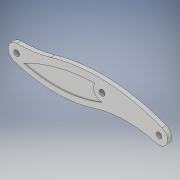
# Autodesk Inventor part: legB_mini
Saved by Autodesk Inventor 2017 (Build 210142000, 142)
## iProperties
Created: 2016-08-26
Part Number: legB_mini
Material: Generic
Document SubType Name: Modeling
Designer: Nic
Density: 1 g/cm^3
Appearance: Default
Author: Nic
Autodesk Inventor part; units mm, degrees
ref_plane "YZ Plane" through (0, 0, 0) normal (1, 0, 0) x (0, 1, 0)
ref_plane "XZ Plane" through (0, 0, 0) normal (0, 1, 0) x (-1, 0, 0)
sketch "Sketch1" plane through (0, 0, 0) normal (0, 0, 1) x (1, 0, 0)
  circle A0 centre (0, 0) radius 1
  circle A1 centre (50, 0) radius 1
  circle A2 centre (30, 3) radius 1
  circle A3 centre (0, 0) radius 3 construction
  circle A4 centre (50, 0) radius 3 construction
  circle A5 centre (30, 3) radius 3 construction
  arc A6 (0, 3) -> (-0.9702, -2.8388) centre (0, 0) ccw
  arc A7 (-0.9702, -2.8388) -> (27.1592, -3.1605) centre (13.5833, 39.7428) ccw
  arc A8 (51.1182, 2.7838) -> (11.9578, 4.708) centre (28.755, -52.8928) ccw
  arc A9 (0, 3) -> (11.9578, 4.708) centre (0, 45.7132) ccw
  arc A10 (49.1676, -2.8822) -> (27.1592, -3.1605) centre (38.6233, -39.39) ccw
  arc A11 (49.1676, -2.8822) -> (51.1182, 2.7838) centre (50, 0) ccw
  arc A12 (27.4576, 4.5925) -> (2.414, -1.7812) centre (28.755, -52.8928) ccw
  arc A13 (2.414, -1.7812) -> (30, 0) centre (13.5833, 39.7428) ccw
  arc A14 (27.4576, 4.5925) -> (30, 0) centre (30, 3) ccw
  dimension "d6" = 6
  dimension "d0" = 2
  dimension "d1" = 2
  dimension "d2" = 2
  dimension "d3" = 50
  dimension "d4" = 3
  dimension "d5" = 30
  dimension "d7" = 6
  dimension "d8" = 6
  dimension "d35" = 3
  dimension "d58" = 3
  dimension "d63" = 2
  dimension "d64" = 2.5
  dimension "d65" = 45
  dimension "d66" = 38
  dimension "d67" = 60
  constraints: 20 point on circle, 14 centre point, 7 coincident, 6 tangent, 2 concentric, 2 vertical alignment, 1 horizontal alignment, 3 other
  measures "d0" diameter of A0
  measures "d1" diameter of A1
  measures "d2" diameter of A2
  measures "d3" distance of A1.centre point (0, 0)
  measures "d4" vertical distance of A1.centre A2.centre
  measures "d5" horizontal distance of point (0, 0) A2.centre
  measures "d7" diameter of A4
  measures "d8" diameter of A5
  measures "d35" radius of A11
  measures "d58" radius of A6
  measures "d63" radial gap between concentric circles of A7 A13
  measures "d64" radial gap between concentric circles of A8 A12
  measures "d65" radius of A7
  measures "d66" radius of A10
  measures "d67" radius of A8
extrude "Extrusion2" add sketch "Sketch1" along normal blind 1.5 contours A9 A8 A11 A10 A7 A6 | A14 A13 A12
extrude "Extrusion3" cut sketch "Sketch1" along normal blind 0.3 contours A14 A13 A12
ref_plane "Work Plane1" through (0, 0, 0.75) normal (0, 0, 1) x (1, 0, 0)
mirror "Mirror1" about plane through (0, 0, 0.75) normal (0, 0, 1) of "Extrusion3"
body "Solid2"
